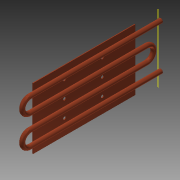
# Autodesk Inventor part: RezLemezHocserelo
Saved by Autodesk Inventor 2015 (Build 190159000, 159)
## iProperties
Created: 2014-11-06
Part Number: RezLemezHocserelo
Material: Copper, Wrought
Document SubType Name: Modeling
Designer: laca
Mass: 224.806 g
Surface Area: 508.631 cm^2
Volume: 25.1461 cm^3
Density: 8.94 g/cm^3
Appearance: Copper - Satin
Author: laca
Autodesk Inventor part; units mm, degrees
ref_plane "YZ Plane" through (0, 0, 0) normal (1, 0, 0) x (0, 1, 0)
ref_plane "XZ Plane" through (0, 0, 0) normal (0, 1, 0) x (-1, 0, 0)
ref_plane "XY Plane" through (0, 0, 0) normal (0, 0, 1) x (1, 0, 0)
derived "HutoBorda.ipt"
sketch "Sketch7" plane through (0, 0, 47.8198) normal (1, 0, 0) x (0, 0, -1)
  circle A0 centre (17, 43) radius 2 projected
  line L0 (68.3948, -121.6906) -> (68.3948, -64.6373) projected
  line L1 (68.3948, -121.6906) -> (33.156, -121.6906) projected
  circle A1 centre (17, 95) radius 2 projected
  circle A2 centre (40, 43) radius 2 projected
  circle A3 centre (40, 95) radius 2 projected
  circle A4 centre (63, 43) radius 2 projected
  circle A5 centre (63, 95) radius 2 projected
  line L2 (0, 0) -> (0, 140) projected
  line L3 (0, 0) -> (84, 0) projected
  line L4 (0, 0) -> (84, 0)
  line L5 (84, 0) -> (84, 140)
  line L6 (84, 140) -> (0, 140)
  line L7 (0, 140) -> (0, 0)
  line L8 (20, 168) -> (20, 168)
  line L9 (40, -12) -> (40, -12)
  line L10 (60, 168) -> (60, 168)
  point P0 (47.8198, 0)
  dimension "d34" = 140
  constraints: 14 end point, 2 horizontal, 2 parallel, 1 perpendicular, 1 vertical
  measures "d34" distance of L4.end L5.end
extrude "Extrusion1" add sketch "Sketch7" along normal blind 1
sketch "Sketch4" plane through (0, 0, 47.8198) normal (-1, 0, 0) x (0, 0, 1)
  line L0 (-10, 171.9161) -> (-10, -8.0839)
  line L1 (-30, 151.9161) -> (-30, -8.0839)
  line L2 (-50, 151.9161) -> (-50, -8.0839)
  arc A0 (-30, -8.0839) -> (-10, -8.0839) centre (-20, -8.0839) ccw
  arc A1 (-30, 151.9161) -> (-50, 151.9161) centre (-40, 151.9161) ccw
  line L3 (-70, 171.9161) -> (-70, -8.0839)
  arc A2 (-70, -8.0839) -> (-50, -8.0839) centre (-60, -8.0839) ccw
  line L4 (0, 140) -> (0, 0) projected
  line L5 (0, 0) -> (-84, 0) projected
  point P0 (-47.8198, 0)
  dimension "d21" = 180
  dimension "d22" = 20
  dimension "d23" = 20
  dimension "d25" = 20
  dimension "d33" = 10
  dimension "d35" = 8.0838
  dimension "d36" = 160
  dimension "d37" = 180
  constraints: 8 end point, 6 point on circle, 6 tangent, 4 vertical, 3 centre point, 2 horizontal alignment
  measures "d21" distance of L0.start L0.end
  measures "d22" distance between parallel lines of L1 L0
  measures "d23" distance from line of L2.end L1
  measures "d25" distance between parallel lines of L3 L2
  measures "d33" distance between parallel lines of L0 L4
  measures "d35" distance from line of L5 A0.centre
  measures "d36" distance of L1.start L1.end
  measures "d37" distance of L3.start L3.end
ref_plane "Work Plane1" through (0, 171.9161, 37.8198) normal (0, 1, 0) x (1, 0, 0)
sketch "Sketch5" plane through (0, 171.9161, 37.8198) normal (0, 1, 0) x (1, 0, 0)
  circle A0 centre (4, 0.013) radius 2
  circle A1 centre (4, 0.013) radius 3
  line L0 (0, 74) -> (0, -10) projected
  line L1 (1, -10) -> (1, 74) projected
  line L2 (1, 0.013) -> (1, 5.013)
  line L3 (1, 0.013) -> (1, -4.987)
  line L4 (1, -4.987) -> (4, -2.987)
  line L5 (1, 5.013) -> (4, 3.013)
  point P0 (0, 37.8198)
  dimension "d28" = 4
  dimension "d29" = 6
  dimension "d32" = 4
  dimension "d38" = 5
  dimension "d40" = 5
  constraints: 8 end point, 3 point on circle, 3 point on line, 2 centre point, 1 coincident
  measures "d28" diameter of A0
  measures "d29" diameter of A1
  measures "d32" distance from line of L0 A0.centre
  measures "d38" distance of L2.start L2.end
  measures "d40" distance of L2.start L3.end
sweep "Sweep2" add profiles "Sketch5" path "Sketch4" path curves L0 A0 L1 A1 L2 A2 L3 contours A1
equation "\"d23\" = d22"
equation "\"d25\" = d23"
equation "\"d37\" = d21"
body "Solid1"
